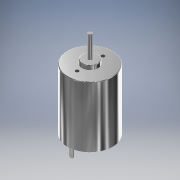
# Autodesk Inventor part: RS-380
Saved by Autodesk Inventor 2020 (Build 240168000, 168)
## iProperties
Created: 2015-02-03
Part Number: RS-380
Material: 一般
Document SubType Name: Modeling
Designer: Riku
Mass: 80 g
Surface Area: 51.5496 cm^2
Volume: 25.7642 cm^3
Density: 3.10378 g/cm^3
Appearance: クローム - つや出し
Author: Riku
Autodesk Inventor part; units mm, degrees
ref_plane "YZ Plane" through (0, 0, 0) normal (1, 0, 0) x (0, 1, 0)
ref_plane "XZ Plane" through (0, 0, 0) normal (0, 1, 0) x (-1, 0, 0)
ref_plane "XY Plane" through (0, 0, 0) normal (0, 0, 1) x (1, 0, 0)
sketch "スケッチ1" plane through (0, 0, 0) normal (0, 0, 1) x (1, 0, 0)
  circle A0 centre (0, 0) radius 14
  dimension "d0" = 28
  constraints: 1 centre point, 1 coincident
  measures "d0" diameter of A0
extrude "押し出し1" add sketch "スケッチ1" along normal blind 37.8
sketch "スケッチ2" plane through (0, 0, 37.8) normal (0, 0, 1) x (1, 0, 0)
  circle A0 centre (0, 0) radius 5
  dimension "d3" = 10
  constraints: 1 centre point, 1 coincident
  measures "d3" diameter of A0
extrude "押し出し2" add sketch "スケッチ2" along normal blind 2.6
sketch "スケッチ3" plane through (0, 0, 40.4) normal (0, 0, 1) x (1, 0, 0)
  circle A0 centre (0, 0) radius 1.15
  dimension "d6" = 2.3
  constraints: 1 centre point, 1 coincident
  measures "d6" diameter of A0
extrude "押し出し3" add sketch "スケッチ3" along normal blind 13.8
sketch "スケッチ4" plane through (0, 0, 0) normal (0, 0, -1) x (-1, 0, 0)
  circle A0 centre (0, 0) radius 1.15 projected
  circle A1 centre (0, 0) radius 5
  dimension "d9" = 10
  constraints: 1 centre point, 1 coincident
  measures "d9" diameter of A1
extrude "押し出し4" add sketch "スケッチ4" along normal blind 2.6 contours A0 | A1
sketch "スケッチ5" plane through (0, 0, 0) normal (0, 0, -1) x (-1, 0, 0)
  line L0 (1.4, -11.7) -> (-1.4, -11.7)
  line L1 (-1.4, -11.7) -> (-1.4, -11.3)
  line L2 (-1.4, -11.3) -> (1.4, -11.3)
  line L3 (1.4, -11.3) -> (1.4, -11.7)
  line L4 (1.4, 11.3) -> (-1.4, 11.3)
  line L5 (-1.4, 11.3) -> (-1.4, 11.7)
  line L6 (-1.4, 11.7) -> (1.4, 11.7)
  line L7 (1.4, 11.7) -> (1.4, 11.3)
  line L8 (0, 0) -> (0, -11.3)
  circle A0 centre (0, 0) radius 1.15 projected
  line L9 (0, 0) -> (0, 11.3)
  dimension "d12" = 2.8
  dimension "d13" = 0.4
  dimension "d14" = 22.6
  dimension "d15" = 1.4
  constraints: 20 end point, 4 parallel, 3 equal length, 3 perpendicular, 2 horizontal, 2 midpoint, 2 point on line, 1 vertical alignment
  measures "d12" distance of L0.start L0.end
  measures "d13" distance of L2.end L0.start
  measures "d14" distance between parallel lines of L4 L2
  measures "d15" distance between parallel lines of L3 L8
extrude "押し出し5" add sketch "スケッチ5" along normal blind 7 contours L4 L5 L6 L7 | L0 L1 L2 L3
fillet "フィレット1" radius 0.5 1 edges at (-14, 0, 37.8)
fillet "フィレット2" radius 0.2 1 edges at (-1.15, 0, 54.2)
fillet "フィレット3" radius 0.5 1 edges at (-5, 0, 40.4)
fillet "フィレット4" radius 0.5 1 edges at (5, 0, -2.6)
fillet "フィレット5" radius 1 1 edges at (-1.4, -11.5, -7)
fillet "フィレット6" radius 1 1 edges at (1.4, -11.5, -7)
fillet "フィレット7" radius 1 1 edges at (-1.4, 11.5, -7)
fillet "フィレット8" radius 1 1 edges at (1.4, 11.5, -7)
fillet "フィレット9" radius 0.2 1 edges at (-14, 0, 0)
sketch "スケッチ6" plane through (0, 0, 37.8) normal (0, 0, 1) x (1, 0, 0)
  circle A0 centre (0, 0) radius 8
  point P0 (0, 8)
  point P1 (0, -8)
  dimension "d27" = 16
  constraints: 2 point on circle, 1 centre point, 1 coincident
  measures "d27" diameter of A0
hole "穴1" at (0, 8, 37.8) at (0, -8, 37.8) direction (0, 0, -1) diameter 2.113 depth 3 thread size "M2.6x0.45" class "6H" standard "ISO Metric profile"
